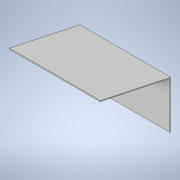
# Autodesk Inventor part: suspensionprotection2
Saved by Autodesk Inventor 2021 (Build 250183000, 183)
## iProperties
Created: 2020-10-26
Part Number: suspensionprotection2
Material: Generic
Document SubType Name: Modeling
Designer: mackeycj
Density: 1 g/cm^3
Appearance: Default
Author: mackeycj
Autodesk Inventor part; units mm, degrees
ref_plane "YZ Plane" through (0, 0, 0) normal (1, 0, 0) x (0, 1, 0)
ref_plane "XZ Plane" through (0, 0, 0) normal (0, 1, 0) x (-1, 0, 0)
ref_plane "XY Plane" through (0, 0, 0) normal (0, 0, 1) x (1, 0, 0)
sketch "Sketch1" plane through (0, 0, 0) normal (1, 0, 0) x (0, 1, 0)
  line L0 (0, 0) -> (158.75, 0)
  line L1 (158.75, 0) -> (158.75, -3.175)
  line L2 (158.75, -3.175) -> (0, -3.175)
  line L3 (0, -3.175) -> (0, 0)
  line L4 (158.75, -3.175) -> (208.9191, 232.852)
  line L5 (158.75, -3.175) -> (400.05, -3.175) construction
  line L6 (208.9191, 232.852) -> (205.8135, 233.5121)
  line L7 (158.75, -3.175) -> (155.6444, -2.5149)
  line L8 (155.6444, -2.5149) -> (205.8135, 233.5121)
  point P0 (156.1789, 0)
  dimension "d0" = 158.75
  dimension "d1" = 3.175
  dimension "d2" = 241.3
  dimension "d3" = 78
  dimension "d4" = 3.175
  dimension "d5" = 3.175
  constraints: 18 end point, 3 perpendicular, 2 horizontal, 2 parallel, 1 equal length
  measures "d0" distance of L1.end L2.end
  measures "d1" distance of L0.end L1.end
  measures "d2" distance of L1.end L4.end
  measures "d3" angle of L5 L4
  measures "d4" distance of L4.end L6.end
  measures "d5" distance of L1.end L7.end
extrude "Extrusion1" add sketch "Sketch1" along normal blind 304.8
body "Solid1"
